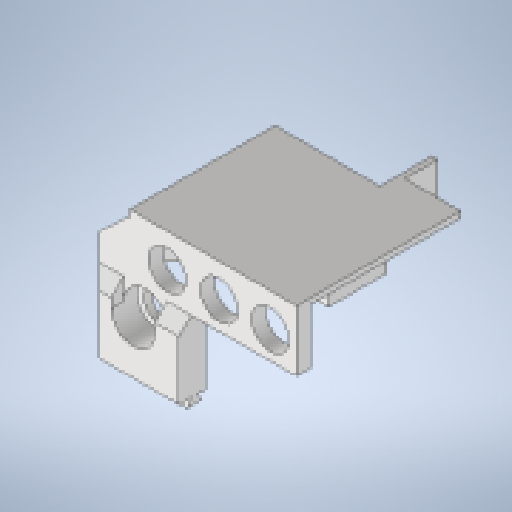
# Autodesk Inventor part: FrontLeftCover
Saved by Autodesk Inventor 2025.1 (Build 291241000, 241)
## iProperties
Created: 2026-04-16
Part Number: FrontLeftCover
Material: Generic
Document SubType Name: Modeling
Designer: User
Density: 1 g/cm^3
Appearance: Default
Author: User
## iProperties of the stored document FrontLeftCover_3DPrint.ipt
Created: 2026-04-17
Part Number: FrontLeftCover_3DPrint
Material: Generic
Document SubType Name: Modeling
Designer: User
Density: 1 g/cm^3
Appearance: Default
Author: User
Autodesk Inventor part; units mm, degrees
sketch "Sketch1" plane through (0, 0, 0) normal (0, 0, 1) x (1, 0, 0)
  line L0 (185.7556, 3.5) -> (29.0886, 3.5) projected
  line L1 (185.7556, 3.731) -> (29.0886, 3.731)
  line L2 (67.9918, 33.5) -> (67.9918, 28.504) projected
  line L3 (143.9918, 33.5) -> (67.9918, 33.5) projected
  line L4 (67.7918, 3.5) -> (67.7918, 33.7)
  line L5 (67.7918, 33.7) -> (143.9918, 33.7)
  line L6 (34.0886, 3.5) -> (34.0886, 0) projected
  line L7 (51.5977, 51.9) -> (63.6977, 51.9) projected
  line L8 (51.5977, 56.9) -> (63.6977, 56.9)
  line L9 (107.2766, 51.9) -> (107.2766, 38.5) projected
  line L10 (112.2766, 51.9) -> (112.2766, 38.5)
  line L11 (112.2766, 33.7) -> (112.2766, 56.9)
  line L12 (112.2766, 56.9) -> (34.0886, 56.9)
  line L13 (34.0886, 56.9) -> (34.0886, 3.731)
  line L14 (34.0886, 56.9) -> (29.0886, 56.9)
  line L15 (29.0886, 56.9) -> (29.0886, 3.731)
  circle A0 centre (57.6477, 45.2) radius 7.9 projected
  circle A1 centre (79.5677, 45.2) radius 7.9 projected
  circle A2 centre (101.2266, 45.2) radius 7.9 projected
  circle A3 centre (57.6477, 45.2) radius 8
  circle A4 centre (79.5677, 45.2) radius 8
  circle A5 centre (101.2266, 45.2) radius 8
  point P0 (0, 0)
  point P1 (29.0886, 3.5)
  point P2 (67.7918, 3.731)
  dimension "d0" = 0.231
  dimension "d1" = 0.2
  dimension "d2" = 5
  dimension "d3" = 5
  dimension "d4" = 0.1
  dimension "d5" = 0.1
  dimension "d6" = 0.1
  constraints: 20 end point, 5 point on line, 3 centre point, 2 parallel, 2 perpendicular, 1 horizontal, 2 other
  measures "d1" distance between parallel lines of L2 L4
  measures "d2" distance between parallel lines of L7 L8
  measures "d3" distance between parallel lines of L9 L10
  measures "d4" radial gap between concentric circles of A0 A3
  measures "d5" radial gap between concentric circles of A1 A4
  measures "d6" radial gap between concentric circles of A2 A5
ref_plane "Work Plane1" through (129.9918, 31.5, -11.1965) normal (0, 0, -1) x (0, 1, 0)
extrude "Extrusion1" add sketch "Sketch1" against normal up to surface (11.1965 mm away) contours L13 L12 L8 L11 L10 L5 L4 L1 | L1 L15 L14 L13
sketch "Sketch2" plane through (0, 0, 0) normal (0, 0, 1) x (1, 0, 0)
  circle A0 centre (57.6477, 45.2) radius 8 projected
  circle A1 centre (79.5677, 45.2) radius 8 projected
  circle A2 centre (101.2266, 45.2) radius 8 projected
  line L0 (112.2766, 56.9) -> (29.0886, 56.9) projected
  line L1 (112.2766, 33.7) -> (112.2766, 56.9) projected
  line L2 (67.7918, 33.7) -> (112.2766, 33.7) projected
  line L3 (29.0886, 56.9) -> (29.0886, 3.731) projected
  line L4 (67.7918, 3.731) -> (67.7918, 33.7) projected
  line L5 (112.2766, 56.9) -> (29.0886, 56.9)
  line L6 (29.0886, 56.9) -> (29.0886, 33.7)
  line L7 (29.0886, 33.7) -> (112.2766, 33.7)
  line L8 (112.2766, 33.7) -> (112.2766, 56.9)
  point P0 (0, 0)
  constraints: 8 end point, 2 parallel, 2 point on line, 1 horizontal, 1 perpendicular
ref_plane "Work Plane2" through (70.7677, 36.4, -5.1965) normal (0, 0, -1) x (0, 1, 0)
extrude "Extrusion2" cut sketch "Sketch2" against normal up to surface (5.1965 mm away)
sketch "Sketch3" plane through (0, 0, 0) normal (0, 0, 1) x (1, 0, 0)
  line L0 (67.7918, 33.7) -> (29.0886, 33.7) projected
  line L1 (29.0886, 33.7) -> (29.0886, 3.731) projected
  line L2 (29.0886, 3.731) -> (67.7918, 3.731) projected
  line L3 (67.7918, 3.731) -> (67.7918, 33.7) projected
  line L4 (34.0886, 28.7) -> (62.7918, 28.7)
  line L5 (62.7918, 28.7) -> (62.7918, 8.731)
  line L6 (62.7918, 8.731) -> (34.0886, 8.731)
  line L7 (34.0886, 8.731) -> (34.0886, 28.7)
  line L8 (48.4402, 24.5) -> (48.4402, 33.5)
  line L9 (29.0886, 33.7) -> (67.7918, 33.7) projected
  line L10 (29.0886, 33.7) -> (29.0886, 56.9) projected
  line L11 (48.4402, 33.7) -> (29.0886, 33.7)
  circle A0 centre (48.4402, 24.5) radius 9.2
  line L12 (48.4402, 33.5) -> (48.4402, 33.7)
  point P0 (0, 0)
  dimension "d11" = 5
  constraints: 14 end point, 2 vertical, 1 horizontal, 1 midpoint, 1 vertical alignment, 5 other
  measures "d11" distance between parallel lines of L0 L4
extrude "Extrusion3" cut sketch "Sketch3" against normal blind 11 contours A0 L4 L8 L12 | L12 L8 L4 A0 | A0 L4
sketch "Sketch4" plane through (112.2766, 56.9, -11.1965) normal (0, 0, -1) x (-1, 0, 0)
  circle A0 centre (63.8364, -32.4) radius 9.2 projected
  circle A1 centre (63.8364, -32.4) radius 6.5
  point P0 (112.2766, -56.9)
  dimension "d16" = 13
  constraints: 1 centre point, 1 coincident
  measures "d16" diameter of A1
extrude "Extrusion4" cut sketch "Sketch4" against normal blind 11 contours A1
sketch "Sketch5" plane through (112.2766, 56.9, -11.1965) normal (0, 0, -1) x (-1, 0, 0)
  circle A0 centre (63.8364, -32.4) radius 9.2 projected
  circle A1 centre (63.8364, -32.4) radius 6.5 projected
  point P0 (112.2766, -56.9)
  point P1 (63.8364, -23.2)
  constraints: 1 vertical alignment
extrude "Extrusion5" add sketch "Sketch5" along normal blind 3
sketch "Sketch6" plane through (0, 0, 0) normal (0, 0, 1) x (1, 0, 0)
  line L0 (48.4402, 33.7) -> (29.0886, 33.7) projected
  line L1 (67.7918, 33.7) -> (48.4402, 33.7) projected
  circle A0 centre (48.4402, 24.5) radius 9.2 projected
  line L2 (39.2402, 24.5) -> (39.2402, 33.7)
  line L3 (57.6402, 24.5) -> (57.6402, 33.7)
  point P0 (0, 0)
  constraints: 4 end point, 2 perpendicular, 2 point on circle, 2 point on line, 2 tangent
extrude "Extrusion6" cut sketch "Sketch6" against normal up to surface (5.1965 mm away) contours A0 L2 L0 | L1 L3 A0
chamfer "Chamfer2" distance 5.196 angle 45 2 edges at (34.1644, 33.7, 0) (62.716, 33.7, 0)
sketch "Sketch7" plane through (29.0886, 56.9, -11.1965) normal (0, 1, 0) x (1, 0, 0)
  line L0 (-29.0886, 22.8921) -> (-3, -3.1965) projected
  line L1 (0, -6.1965) -> (5, -11.1965) projected
  line L2 (2, -8.1965) -> (-5, -1.1965) projected
  line L3 (0, -11.1965) -> (10.1516, -11.1965) projected
  line L4 (0, -6.0005) -> (0, -11.1965) projected
  point P0 (-29.0886, -11.1965)
extrude "Extrusion7" cut sketch "Sketch7" against normal through all
sketch "Sketch8" plane through (29.0886, 3.731, -5) normal (-0.7071068, 0, 0.7071068) x (0.7071068, 0, 0.7071068)
  line L0 (7.0711, 24.773) -> (7.0711, 0) projected
  line L1 (7.0711, 0) -> (0, 0) projected
  line L2 (-41.1375, -3.731) -> (-41.1375, -0.231) projected
  line L3 (-52.5923, 2.269) -> (-42.7639, 2.269) projected
  line L4 (7.0711, 0) -> (30.9028, 0) projected
  line L5 (7.0711, 0) -> (-41.1375, 0)
  line L6 (-0.1389, 29.969) -> (-0.1389, 53.169) projected
  line L7 (-41.1375, 0) -> (-41.1375, 53.169)
  line L8 (-41.1375, 0) -> (12.0315, 0) construction
  line L9 (-41.1375, 53.169) -> (-0.1389, 53.169)
  line L10 (0, 29.773) -> (7.0711, 24.773) projected
  line L11 (-0.1386, 29.969) -> (0, 29.773) projected
  line L12 (-0.1386, 29.969) -> (-0.1389, 29.969) projected
  point P0 (-17.0332, -3.731)
  dimension "d31" = 90
  constraints: 8 end point, 2 horizontal, 2 perpendicular
  measures "d31" angle of L8 L7
extrude "Extrusion8" add sketch "Sketch8" against normal blind 5
sketch "Sketch9" plane through (0, 0, 0) normal (0, 0, 1) x (1, 0, 0)
  line L0 (28.9904, 56.9) -> (29.0886, 56.9) projected
  line L1 (28.9904, 56.9) -> (0, 56.9) projected
  line L2 (29.0886, 56.9) -> (112.2766, 56.9) projected
  circle A0 centre (57.6477, 45.2) radius 8.8 projected
  line L3 (0, 56.9) -> (0, 3.731) projected
  line L4 (0, 3.731) -> (34.0886, 3.731) projected
  line L5 (46.8477, 49.725) -> (46.8477, 40.675) projected
  line L6 (41.8477, 49.725) -> (41.8477, 40.675)
  line L7 (41.8477, 40.675) -> (41.8477, 56.9)
  line L8 (0, 3.731) -> (0, 6.731)
  line L9 (0, 6.731) -> (41.8477, 56.9)
  point P0 (0, 0)
  dimension "d34" = 5
  dimension "d35" = 3
  constraints: 8 end point, 2 point on line, 1 parallel, 1 vertical
  measures "d34" distance between parallel lines of L5 L6
  measures "d35" distance of L3.end L8.end
extrude "Extrusion9" cut sketch "Sketch9" against normal through all contours L0 L2 L9 L3 L1
sketch "Sketch12" plane through (67.7918, 3.731, -11.1965) normal (0, -1, 0) x (1, 0, 0)
  line L0 (-67.7918, -22.8921) -> (-64.2563, -26.4276) projected
  line L1 (-25.7956, -67.1884) -> (-67.7438, -25.2402) projected
  line L2 (-67.7438, -25.2402) -> (-63.0689, -25.2402)
  line L3 (-64.2563, -26.4276) -> (-37.8286, 0) projected
  line L4 (-67.7438, -25.2402) -> (-63.0689, -25.2402) construction
  line L5 (-68.1066, -24.2402) -> (-62.1095, -24.2402)
  line L6 (-62.5423, -24.2402) -> (-62.0689, -24.2402)
  point P0 (-67.7918, 11.1965)
  point P1 (-66.4437, -24.2402)
  dimension "d43" = 1
  constraints: 8 end point, 4 point on line, 2 horizontal, 1 collinear, 1 parallel
  measures "d43" distance between parallel lines of L5 L2
extrude "Extrusion10" cut sketch "Sketch12" against normal blind 10
sketch "Sketch13" plane through (0, 3.731, -34.0886) normal (-0.7071068, 0, -0.7071068) x (-0.7071068, 0, 0.7071068)
  line L0 (-1.9065, 4.6162) -> (-1.9065, 0) projected
  line L1 (0, 3) -> (0, 0) projected
  line L2 (0, 3) -> (-1.9065, 4.6162) projected
  line L3 (-11.5227, 2.269) -> (-1.6943, 2.269) projected
  line L4 (-14.3512, 2.269) -> (-11.5227, 2.269) projected
  line L5 (-14.3512, 2.269) -> (-57.8759, 2.269) projected
  line L6 (-57.8759, 3.269) -> (-14.3512, 3.269)
  line L7 (-14.3512, 3.269) -> (-11.5227, 3.269)
  line L8 (-11.5227, 3.269) -> (-1.6943, 3.269)
  line L9 (-57.8759, 5.769) -> (-14.3512, 5.769)
  line L10 (-14.3512, 5.769) -> (-11.5227, 5.769)
  line L11 (-11.5227, 5.769) -> (-1.6943, 5.769)
  line L12 (0, 37.755) -> (0, 3) projected
  line L13 (-1.6943, 5.769) -> (0, 5.769)
  line L14 (-1.6943, 3.269) -> (0, 3.269)
  line L15 (-46.8759, 2.269) -> (-46.8759, 6.269) projected
  line L16 (-45.8759, 2.269) -> (-45.8759, 6.269)
  point P0 (24.1043, -3.731)
  point P1 (-1.9065, 3.269)
  point P2 (-0.3173, 3.269)
  point P3 (-45.8759, 5.769)
  point P4 (-45.8759, 3.269)
  dimension "d46" = 1
  dimension "d47" = 2.5
  dimension "d48" = 1
  constraints: 18 end point, 2 perpendicular, 2 point on line, 1 parallel, 4 other
  measures "d46" distance between parallel lines of L5 L6
  measures "d47" distance between parallel lines of L6 L9
  measures "d48" distance between parallel lines of L15 L16
extrude "Extrusion11" add sketch "Sketch13" against normal blind 2.5 contours L0 L8 L7 L6 L16 L9 L10 L11 L13 L12 L14 L2
sketch "Sketch14" plane through (2.3097, 9.5, -35.4367) normal (0, 1, 0) x (1, 0, 0)
  line L0 (-2.3097, -1.3481) -> (30.1294, 31.091) projected
  line L1 (65.6821, 17.6568) -> (65.6821, 49.3641) projected
  line L2 (64.6821, 17.6568) -> (64.6821, 49.3641)
  line L3 (30.1294, 31.091) -> (64.6821, 31.091)
  line L4 (30.1294, 31.091) -> (64.6821, 31.091) construction
  line L5 (64.6821, 31.091) -> (64.6821, 28.591)
  line L6 (64.6821, 28.591) -> (27.6294, 28.591)
  point P0 (-2.3097, -35.4367)
  dimension "d51" = 1
  dimension "d52" = 0
  dimension "d53" = 2.5
  constraints: 10 end point, 3 point on line, 1 collinear, 1 horizontal, 1 parallel, 1 perpendicular
  measures "d51" distance between parallel lines of L1 L2
  measures "d52" distance between parallel lines of L3 L4
  measures "d53" distance of L4.end L5.end
extrude "Extrusion12" add sketch "Sketch14" against normal up to surface (2.5 mm away)
sketch "Sketch15" plane through (66.9918, 9.5, -66.5277) normal (0, 0, -1) x (-1, 0, 0)
  line L0 (0, 0) -> (0, -2.5) projected
  line L1 (-0.8, 24.2) -> (-45.2848, 24.2) projected
  line L2 (-0.8, 25.2) -> (-45.2848, 25.2)
  line L3 (0, -2.5) -> (0, 25.2)
  line L4 (0, 25.2) -> (-0.8, 25.2)
  line L5 (-23.6095, 43.606) -> (-23.6095, 36.106) projected
  line L6 (-21.6095, 43.606) -> (-21.6095, 36.106)
  line L7 (-26.6095, 55.106) -> (-23.6095, 55.106) projected
  line L8 (-26.6095, 57.106) -> (-23.6095, 57.106)
  line L9 (-21.6095, 25.2) -> (-21.6095, 57.106)
  line L10 (61.2689, -5.769) -> (61.2689, 4.092) projected
  line L11 (-21.6095, 57.106) -> (61.2689, 4.092)
  line L12 (34.5877, 0) -> (55.7465, 0) construction
  line L13 (0, 0) -> (34.5527, 0) projected
  line L14 (34.5527, 0) -> (34.5527, 21.1812)
  line L15 (34.5527, 0) -> (55.7339, 0) construction
  point P0 (66.9918, -9.5)
  point P1 (-21.6095, 43.606)
  point P2 (-21.6095, 36.106)
  dimension "d56" = 1
  dimension "d57" = 2
  dimension "d58" = 2
  dimension "d60" = 90
  constraints: 20 end point, 3 parallel, 2 horizontal, 2 perpendicular, 2 point on line, 2 vertical
  measures "d56" distance between parallel lines of L1 L2
  measures "d57" distance between parallel lines of L5 L6
  measures "d58" distance between parallel lines of L7 L8
  measures "d60" angle of L15 L14
extrude "Extrusion13" add sketch "Sketch15" against normal blind 2.5
sketch "Sketch16" plane through (0, 3.731, -34.0886) normal (-0.7071068, 0, -0.7071068) x (-0.7071068, 0, 0.7071068)
  line L0 (-45.8759, 5.769) -> (-45.8759, 26.9502) projected
  line L1 (-5, 9.861) -> (-2.5865, 5.769) projected
  line L2 (0, 5.769) -> (-45.8759, 5.769) projected
  line L3 (-45.8759, 26.9502) -> (-5, 9.861)
  point P0 (24.1043, -3.731)
  constraints: 2 end point
extrude "Extrusion14" add sketch "Sketch16" against normal blind 2.5
ref_plane "Work Plane3" through (41.8477, 56.9, -5.1965) normal (0.6694405, -0.7146449, 0.2028105) x (-0.6019698, -0.6818384, -0.4156065)
sketch "Sketch18" plane through (41.8477, 56.9, -5.1965) normal (0.6694405, -0.7146449, 0.2028105) x (-0.6019698, -0.6818384, -0.4156065)
  line L0 (71.2225, -0.3903) -> (69.5179, 0) projected
  line L1 (49.0303, 46.1898) -> (69.5179, 0)
  line L2 (69.5179, 0) -> (0, 0)
  line L3 (49.0303, 46.1898) -> (-9.2725, 76.2461) projected
  line L4 (0, 0) -> (49.0303, 46.1898)
  point P0 (61.828, -31.7078)
  constraints: 6 end point, 1 horizontal
extrude "Extrusion15" add sketch "Sketch18" along normal blind 2.5
sketch "Sketch19" plane through (0, 9.5, -34.0886) normal (-0.4352951, -0.156138, 0.8866449) x (0.6019698, 0.6818384, 0.4156065)
  line L0 (1.5874, 0) -> (3.449, 1.2745) projected
  line L1 (3.449, 1.2745) -> (4.9358, 0) projected
  line L2 (3.449, 1.2745) -> (20.4876, 0) projected
  line L3 (69.5179, 0) -> (0, 0) projected
  line L4 (57.8032, 0) -> (67.0243, 1.2169) projected
  line L5 (67.0243, 1.2169) -> (69.5179, 0) projected
  point P0 (7.69, -13.7027)
extrude "Extrusion16" cut sketch "Sketch19" against normal through all
sketch "Sketch20" plane through (0, 9.5, -34.0886) normal (-0.4352951, -0.156138, 0.8866449) x (0.6019698, 0.6818384, 0.4156065)
  line L0 (31.6827, -2.5) -> (35.7207, -0.8873) projected
  line L1 (53.8612, -2.5) -> (31.6827, -2.5) projected
  line L2 (54.8939, -0.3839) -> (53.8612, -2.5) projected
  line L3 (69.5179, 0) -> (54.8939, -0.3839) projected
  line L4 (69.5179, 0) -> (0, 0) projected
  line L5 (1.8617, -1.7762) -> (0, 0) projected
  line L6 (35.7207, -0.8873) -> (1.8617, -1.7762) projected
  line L7 (51.3092, -2.4282) -> (1.3558, -2.0063) projected
  line L8 (1.7988, -1.5419) -> (1.3558, -2.0063) projected
  point P0 (7.69, -13.7027)
  point P1 (1.7118, -1.6332)
  point P2 (32.2652, -2.2674)
extrude "Extrusion17" add sketch "Sketch20" along normal up to surface surface through (29.0886, 56.9, -5) normal (0.7071068, 0, -0.7071068)
sketch "Sketch21" plane through (112.2766, 56.9, -5.1965) normal (0, 1, 0) x (1, 0, 0)
  line L0 (-70.4289, 0) -> (0, 0) projected
  line L1 (-70.4289, 0) -> (-74.695, -8.6895) projected
  line L2 (-74.695, -8.6895) -> (-112.2766, 28.8921) projected
  line L3 (-62.6289, 0) -> (-46.6289, 0) projected
  line L4 (-83.188, 0) -> (-73.0364, 0) projected
  line L5 (-60.1795, 0) -> (-83.188, 0)
  line L6 (-68.6111, 6) -> (-70.4289, 0) projected
  line L7 (-70.4289, 0) -> (-83.3845, 0)
  point P0 (-112.2766, -5.1965)
  constraints: 4 end point, 3 point on line, 1 horizontal
extrude "Extrusion18" cut sketch "Sketch21" against normal up to surface surface through (91.4796, 31.102, -2.598) normal (0, 0.7071068, 0.7071068)
sketch "Sketch22" plane through (67.7918, 33.7, -5.1965) normal (0, 0, 1) x (1, 0, 0)
  line L0 (-37.436, 11.8978) -> (-36.8153, 10.1671) projected
  line L1 (-25.9441, 23.2) -> (-37.436, 11.8978) projected
  line L2 (-25.9441, 23.2) -> (-36.8153, 10.1671) projected
  point P0 (-67.7918, -33.7)
extrude "Extrusion19" add sketch "Sketch22" against normal up to surface surface through (33.3015, 46.6544, -11.1965) normal (0.6850081, -0.6965045, 0.2136479)
sketch "Sketch23" plane through (112.2766, 56.9, -5.1965) normal (0, 1, 0) x (1, 0, 0)
  line L0 (-70.4289, 0) -> (-68.7553, -0.507) projected
  line L1 (-68.8331, 0) -> (-68.7553, -0.507) projected
  line L2 (-70.4289, 0) -> (0, 0) projected
  point P0 (-112.2766, -5.1965)
extrude "Extrusion20" cut sketch "Sketch23" against normal blind 10
sketch "Sketch24" plane through (112.2766, 56.9, -5.1965) normal (0, 1, 0) x (1, 0, 0)
  line L0 (0, 0) -> (0, 6) projected
  line L1 (-70.4289, 0) -> (0, 0) projected
  line L2 (-38.7589, 41.9) -> (-26.6589, 41.9) projected
  line L3 (-38.7589, 56.9) -> (-26.6589, 56.9)
  line L4 (0, 0) -> (-70.4289, 0)
  line L5 (-79.8375, 61.3312) -> (-23.6753, 61.3312) projected
  line L6 (-70.4289, 0) -> (0, 0)
  line L7 (0, 0) -> (0, 61.3312)
  line L8 (0, 61.3312) -> (-70.4289, 61.3312)
  line L9 (-70.4289, 61.3312) -> (-70.4289, 0)
  point P0 (-112.2766, -5.1965)
  point P1 (-70.4289, 61.3312)
  point P2 (-23.6753, 61.3312)
  dimension "d33" = 0
  dimension "d77" = 15
  constraints: 12 end point, 3 parallel, 2 horizontal, 1 perpendicular
  measures "d77" distance between parallel lines of L2 L3
extrude "Extrusion21" add sketch "Sketch24" along normal blind 2.5
sketch "Sketch25" plane through (66.9918, 7, -66.5277) normal (0, 0, -1) x (-1, 0, 0)
  line L0 (-6.4358, 49.9) -> (25.1441, 49.9) projected
  line L1 (34.5527, 23.6812) -> (-6.4358, 49.9) projected
  line L2 (38.0997, 37.7639) -> (25.1441, 49.9) projected
  line L3 (25.1441, 49.9) -> (22.6441, 49.9)
  line L4 (22.6441, 49.9) -> (22.6441, 31.2987)
  point P0 (66.9918, -7)
  dimension "d80" = 2.5
  constraints: 4 end point, 2 point on line, 1 perpendicular
  measures "d80" distance of L0.end L3.end
extrude "Extrusion22" add sketch "Sketch25" against normal blind 2.5
sketch "Sketch26" plane through (66.9918, 7, -66.5277) normal (0, 0, -1) x (-1, 0, 0)
  line L0 (22.6441, 49.9) -> (25.1441, 49.9) projected
  line L1 (22.6441, 31.2987) -> (22.6441, 49.9) projected
  line L2 (34.5527, 23.6812) -> (22.6441, 31.2987) projected
  line L3 (25.1441, 49.9) -> (25.1441, 52.4) projected
  line L4 (25.1441, 49.9) -> (25.1441, 29.6995)
  point P0 (66.9918, -7)
  constraints: 2 end point, 1 collinear, 1 point on line
extrude "Extrusion23" add sketch "Sketch26" against normal up to surface surface through (32.4391, 30.6812, -66.5277) normal (0.7296167, 0.5811913, -0.3603834)
sketch "Sketch27" plane through (40.9273, 54.335, -11.1965) normal (0.7296167, 0.5811913, -0.3603834) x (-0.1396745, -0.3892292, -0.9104898)
  line L0 (-6.5899, 0) -> (-0.4642, 0) projected
  line L1 (0, 0) -> (-0.4642, 0) projected
  line L2 (60.7709, 0) -> (0, 0) projected
  line L3 (45.3092, 0) -> (60.7709, 0) projected
  line L4 (44.0106, 0) -> (45.3092, 0) projected
  line L5 (-0.0566, 0) -> (44.0106, 0) projected
  line L6 (-0.0566, 0) -> (-6.5899, 0) projected
  line L7 (0.3212, -1.4419) -> (5.3923, -2.5) projected
  line L8 (58.5819, -2.5) -> (5.3923, -2.5) projected
  line L9 (58.1767, -0.6807) -> (58.5819, -2.5) projected
  line L10 (60.7709, 0) -> (58.1767, -0.6807) projected
  line L11 (60.7709, 0) -> (0, 0) projected
  line L12 (0.3212, -1.4419) -> (0, 0) projected
  line L13 (-6.5899, 0) -> (-0.4642, 0) projected
  line L14 (-0.4642, 0) -> (0.3212, -1.4419) projected
  point P0 (16.671, -13.7027)
  point P1 (60.7709, 0)
extrude "Extrusion24" add sketch "Sketch27" along normal blind 14.5
sketch "Sketch28" plane through (43.5213, 55.1134, -4.6895) normal (0.6694405, -0.7146449, 0.2028105) x (0.6019698, 0.6818384, 0.4156065)
  line L0 (-38.2241, -49.0084) -> (-27.3128, -25.7305) projected
  line L1 (-27.3128, -25.7305) -> (-21.5421, -20.2941) projected
  line L2 (-21.5421, -20.2941) -> (-5.6654, -5.3372) projected
  line L3 (-35.118, -50.4632) -> (-6.372, -10.7103) projected
  line L4 (-35.6288, -50.3463) -> (-38.2241, -49.0084) projected
  line L5 (-23.1287, -8.3115) -> (-2.6947, -12.9908) projected
  line L6 (-35.118, -50.4632) -> (-35.6288, -50.3463) projected
  line L7 (-33.3168, -51.3076) -> (-35.118, -50.4632) projected
  line L8 (-38.2464, -48.9969) -> (-48.608, -44.14) projected
  line L9 (-38.2241, -49.0084) -> (-38.2464, -48.9969) projected
  point P0 (-61.828, 31.7078)
  point P1 (-7.2644, -11.9444)
  point P2 (-11.6201, -10.9469)
extrude "Extrusion25" cut sketch "Sketch28" along normal blind 14.5
sketch "Sketch29" plane through (44.3477, 42.2304, -64.0277) normal (1, 0, 0) x (0, 0, -1)
  line L0 (-52.8312, 14.6696) -> (2.5, 14.6696) projected
  line L1 (0, -7.5304) -> (0, 14.6696) projected
  line L2 (-52.8312, -8.5304) -> (-52.8312, 14.6696) projected
  line L3 (-52.8312, 14.6696) -> (0, 14.6696)
  line L4 (0, 14.6696) -> (0, -7.5304)
  line L5 (0, -7.5304) -> (-52.8312, -7.5304)
  line L6 (-52.8312, -7.5304) -> (-52.8312, 14.6696)
  point P0 (-64.0277, -42.2304)
  constraints: 8 end point, 2 parallel, 1 horizontal, 1 perpendicular
extrude "Extrusion26" cut sketch "Sketch29" along normal blind 14.5
sketch "Sketch31" plane through (43.5213, 55.1134, -4.6895) normal (0.6694405, -0.7146449, 0.2028105) x (0.6019698, 0.6818384, 0.4156065)
  line L0 (-7.2644, -11.9444) -> (-10.8274, -11.1285) projected
  line L1 (-10.8274, -11.1285) -> (-11.6201, -10.9469) projected
  line L2 (-8.7215, -8.2163) -> (-11.6201, -10.9469) projected
  line L3 (-8.7215, -8.2163) -> (-5.2019, -4.9006) projected
  line L4 (-0.9887, -6.4081) -> (-22.9457, -53.2507) projected
  line L5 (39.9024, -35.9772) -> (-0.9887, -6.4081) projected
  line L6 (-5.2019, -4.9006) -> (-5.6654, -5.3372) projected
  line L7 (-5.6654, -5.3372) -> (-0.9887, -6.4081) projected
  line L8 (-20.7848, 2.4037) -> (-5.2019, -4.9006) projected
  line L9 (-11.6201, -10.9469) -> (-3.9406, -12.7055)
  line L10 (-3.9406, -12.7055) -> (-0.9887, -6.4081)
  line L11 (-5.2019, -4.9006) -> (-11.6201, -10.9469)
  line L12 (-11.0625, -2.1535) -> (-1.1683, -6.7913)
  point P0 (-61.828, 31.7078)
  point P1 (-1.1683, -6.7913)
  point P2 (-5.2019, -4.9006)
  point P3 (-7.2644, -11.9444)
  point P4 (-3.9406, -12.7055)
  constraints: 8 end point, 3 point on line, 2 collinear
extrude "Extrusion27" cut sketch "Sketch31" against normal up to surface contours L0 L1 L2 L3 L7 L12 L4 L9 | L7 L3 L12 surface through (70.6826, 30.3155, -11.1965) normal (0, 0, -1)
sketch "Sketch32" plane through (112.2766, 59.4, -5.1965) normal (0, 1, 0) x (1, 0, 0)
  line L0 (-34.9406, 61.3312) -> (-70.4289, 61.3312) projected
  line L1 (-59.6181, 61.3312) -> (-88.0349, 61.3312)
  line L2 (-88.0349, 61.3312) -> (-88.0349, 76.9498)
  line L3 (-88.0349, 76.9498) -> (-59.6181, 76.9498)
  line L4 (-59.6181, 76.9498) -> (-59.6181, 61.3312)
  point P0 (-112.2766, -5.1965)
  point P1 (-70.4289, 61.3312)
  constraints: 8 end point, 2 parallel, 1 horizontal, 1 perpendicular, 1 point on line
extrude "Extrusion28" cut sketch "Sketch32" against normal through all
sketch "Sketch33" plane through (66.9918, 7, -66.5277) normal (0, 0, -1) x (-1, 0, 0)
  line L0 (34.5527, 23.6812) -> (28.6733, 28.2363) projected
  line L1 (34.5527, 23.6812) -> (28.2542, 27.7102) projected
  line L2 (28.6733, 28.2363) -> (28.2542, 27.7102) projected
  point P0 (66.9918, -7)
extrude "Extrusion29" add sketch "Sketch33" along normal up to surface surface through (34.4185, 29.7466, -64.0277) normal (-0.2818831, -0.2245398, -0.9328043)
sketch "Sketch34" plane through (112.2766, 59.4, -5.1965) normal (0, 1, 0) x (1, 0, 0)
  line L0 (-70.4289, 0) -> (0, 0) projected
  line L1 (-63.8114, 0) -> (-74.8638, 0)
  line L2 (-74.8638, 0) -> (-74.8638, -8.063)
  line L3 (-74.8638, -8.063) -> (-63.8114, -8.063)
  line L4 (-63.8114, -8.063) -> (-63.8114, 0)
  point P0 (-112.2766, -5.1965)
  point P1 (-70.4289, 0)
  constraints: 8 end point, 2 parallel, 1 horizontal, 1 perpendicular, 1 point on line
extrude "Extrusion30" cut sketch "Sketch34" against normal blind 10
sketch "Sketch35" plane through (41.8477, 39.4947, -66.5277) normal (-1, 0, 0) x (0, 0, 1)
  line L0 (0, 19.9053) -> (61.3312, 19.9053) projected
  line L1 (-10.2184, 45.465) -> (63.5572, 45.465)
  line L2 (63.5572, 45.465) -> (63.5572, 19.9053)
  line L3 (63.5572, 19.9053) -> (-10.2184, 19.9053)
  line L4 (-10.2184, 19.9053) -> (-10.2184, 45.465)
  point P0 (66.5277, -39.4947)
  point P1 (0, 19.9053)
  point P2 (61.3312, 19.9053)
  constraints: 8 end point, 2 parallel, 1 horizontal, 1 perpendicular
extrude "Extrusion31" cut sketch "Sketch35" against normal through all
sketch "Sketch36" plane through (0, 3.731, -34.0886) normal (-0.7071068, 0, -0.7071068) x (-0.7071068, 0, 0.7071068)
  line L0 (-2.5865, 5.769) -> (-3.5544, 7.4101) projected
  line L1 (0, 5.769) -> (-2.5865, 5.769) projected
  line L2 (0, 5.769) -> (-3.5544, 7.4101) projected
  point P0 (24.1043, -3.731)
extrude "Extrusion32" add sketch "Sketch36" against normal up to surface surface through (0, 9.5, -34.0886) normal (-0.3737746, -0.5599702, -0.7394092)
sketch "Sketch37" plane through (0, 3.731, -34.0886) normal (-0.7071068, 0, -0.7071068) x (-0.7071068, 0, 0.7071068)
  line L0 (0, 5.769) -> (-45.8759, 26.9502) projected
  line L1 (-45.8759, 26.9502) -> (-45.8759, 3.269) projected
  line L2 (-45.8759, 3.269) -> (-1.9065, 3.269) projected
  line L3 (-1.9065, 3.269) -> (-1.9065, 0) projected
  line L4 (0, 0) -> (-1.9065, 0) projected
  line L5 (0, 3) -> (0, 0) projected
  line L6 (0, 3) -> (-0.3173, 3.269) projected
  line L7 (-0.3173, 3.269) -> (0, 3.269) projected
  line L8 (0, 3.269) -> (0, 5.769) projected
  line L9 (-0.3173, 3.269) -> (0, 3.269) projected
  line L10 (0, 3.269) -> (0, 3) projected
  point P0 (24.1043, -3.731)
extrude "Extrusion33" add sketch "Sketch37" along normal up to surface contours L10 L6 L7 surface through (41.8477, 56.9, 0) normal (0.7679186, -0.6405475, 0)
chamfer "Chamfer3" distance 3 angle 45 1 edges at (57.6402, 24.5, -11.1965)
sketch "Sketch38" plane through (5.723, 3.731, -35.4367) normal (0, 0, -1) x (-1, 0, 0)
  line L0 (0.8393, 6.4629) -> (0, 7.2491) projected
  line L1 (0, 0) -> (0, 7.2491) projected
  line L2 (0.8393, 3.269) -> (0.8393, 6.4629) projected
  line L3 (4.3749, 3.269) -> (0.8393, 3.269) projected
  line L4 (4.3749, 3.269) -> (0, 3.269)
  line L5 (-26.7162, 3.269) -> (4.3749, 3.269) projected
  point P0 (5.723, -3.731)
  constraints: 2 end point, 2 point on line
extrude "Extrusion34" add sketch "Sketch38" along normal up to surface surface through (17.9873, 8.25, -48.5404) normal (0.7071068, 0, 0.7071068)
sketch "Sketch39" plane through (67.7918, 3.731, -11.1965) normal (1, 0, 0) x (0, 0, -1)
  line L0 (-8.1965, -3.231) -> (-6.1965, -0.231) projected
  line L1 (-1.1965, -3.231) -> (-8.1965, -3.231) projected
  line L2 (-3.1965, -0.231) -> (-1.1965, -3.231) projected
  line L3 (-6.0193, -0.3492) -> (-7.7985, -3.018)
  line L4 (-7.7985, -3.018) -> (-1.5945, -3.018)
  line L5 (-1.5945, -3.018) -> (-3.3737, -0.3492)
  line L6 (-11.1965, 0) -> (0, 0) projected
  line L7 (-7.7985, -3.018) -> (-5.7865, 0)
  line L8 (-1.5945, -3.018) -> (-3.6065, 0)
  point P0 (-11.1965, -3.731)
  point P1 (-3.3737, -0.3492)
  point P2 (-6.0193, -0.3492)
  dimension "d110" = 0.213
  constraints: 10 end point, 4 point on line, 2 other
  measures "d110" distance between parallel lines of L0 L3
extrude "Extrusion35" add sketch "Sketch39" against normal up to surface surface through (29.0886, 56.9, -5) normal (0.7071068, 0, -0.7071068)
sketch "Sketch40" plane through (66.9918, 7, -66.5277) normal (0, 0, -1) x (-1, 0, 0)
  line L0 (-21.6095, 49.9) -> (-21.6095, 27.7) projected
  line L1 (-21.6095, 27.7) -> (0, 27.7) projected
  line L2 (-45.2848, 52.4) -> (25.1441, 52.4) projected
  line L3 (-21.6095, 27.7) -> (-19.1095, 27.7)
  line L4 (-19.1095, 27.7) -> (-19.1095, 52.4)
  line L5 (-19.1095, 52.4) -> (-21.6095, 52.4)
  line L6 (-21.6095, 52.4) -> (-21.6095, 27.7)
  point P0 (66.9918, -7)
  point P1 (-21.6095, 52.4)
  dimension "d113" = 2.5
  constraints: 8 end point, 2 parallel, 1 horizontal, 1 perpendicular, 1 point on line
  measures "d113" distance of L5.end L4.end
ref_plane "Work Plane4" through (94.3013, 43.856, -88.3598) normal (0, 0, -1) x (0, 1, 0)
extrude "Extrusion36" add sketch "Sketch40" along normal up to surface (21.832 mm away)
sketch "Sketch41" plane through (112.2766, 59.4, -5.1965) normal (0, 1, 0) x (1, 0, 0)
  line L0 (-23.6753, 61.3312) -> (-23.6753, 83.1633) projected
  line L1 (0, 61.3312) -> (-23.6753, 61.3312) projected
  line L2 (0, 0) -> (0, 61.3312) projected
  line L3 (-18.5753, 69.2633) -> (66.4247, 69.2633) projected
  line L4 (-23.6753, 61.3312) -> (0, 61.3312)
  line L5 (0, 61.3312) -> (0, 69.2633)
  line L6 (0, 69.2633) -> (-23.6753, 69.2633)
  line L7 (-23.6753, 69.2633) -> (-23.6753, 61.3312)
  point P0 (-112.2766, -5.1965)
  constraints: 8 end point, 2 parallel, 1 horizontal, 1 perpendicular, 1 point on line
extrude "Extrusion37" add sketch "Sketch41" against normal up to surface (2.5 mm away)
sketch "Sketch42" plane through (86.1013, 34.7, -66.5277) normal (-1, 0, 0) x (0, 0, 1)
  line L0 (0, 24.7) -> (0, 0) projected
  line L1 (0, 0) -> (-21.832, 0) projected
  line L2 (-21.832, 24.7) -> (-21.832, 0) projected
  line L3 (2.5, 0) -> (-21.832, 0) projected
  line L4 (-21.832, 0) -> (-21.832, 2.5)
  line L5 (-21.832, 2.5) -> (0, 2.5)
  point P0 (66.5277, -34.7)
  dimension "d118" = 2.5
  constraints: 4 end point, 2 point on line, 1 perpendicular
  measures "d118" distance of L1.end L4.end
extrude "Extrusion38" add sketch "Sketch42" along normal up to surface (19.1095 mm away)
sketch "Sketch43" plane through (66.9918, 34.7, -88.3598) normal (-1, 0, 0) x (0, 0, 1)
  line L0 (21.832, 2.5) -> (0, 2.5) projected
  line L1 (21.832, 0) -> (21.832, -27.7) projected
  line L2 (21.832, 2.5) -> (21.832, 0) projected
  line L3 (21.832, 2.5) -> (0, 2.5)
  line L4 (0, 2.5) -> (0, -27.7)
  line L5 (0, -27.7) -> (21.832, -27.7)
  line L6 (21.832, -27.7) -> (21.832, 2.5)
  point P0 (88.3598, -34.7)
  point P1 (21.832, -27.7)
  constraints: 8 end point, 2 parallel, 1 horizontal, 1 perpendicular
extrude "Extrusion39" add sketch "Sketch43" along normal blind 2.5
sketch "Sketch44" plane through (67.7918, 3.731, -11.1965) normal (1, 0, 0) x (0, 0, -1)
  line L0 (-11.1965, 0) -> (-11.1965, 24.773) projected
  line L1 (-11.1965, -0.231) -> (-6.1965, -0.231) projected
  line L2 (0, 0) -> (0, 29.969) projected
  line L3 (-8.6965, 0) -> (-8.6965, 24.773)
  line L4 (-2.5, 0) -> (-2.5, 29.969)
  line L5 (-8.6965, 24.773) -> (-2.5, 24.773)
  line L6 (-8.6965, 0) -> (-8.6965, 2.5)
  line L7 (-8.6965, 2.5) -> (-2.5, 2.5)
  point P0 (-11.1965, -3.731)
  dimension "d123" = 2.5
  dimension "d124" = 2.5
  dimension "d125" = 2.5
  constraints: 10 end point, 3 point on line, 2 parallel, 2 perpendicular
  measures "d123" distance between parallel lines of L0 L3
  measures "d124" distance between parallel lines of L2 L4
  measures "d125" distance of L3.start L6.end
extrude "Extrusion40" cut sketch "Sketch44" against normal blind 7
sketch "Sketch45" plane through (64.4918, 34.7, -88.3598) normal (-1, 0, 0) x (0, 0, 1)
  line L0 (-5.5815, -24.7) -> (4.4185, -24.7) projected
  line L1 (4.4185, -24.7) -> (19.9749, -24.7) projected
  line L2 (19.9749, -28.7) -> (19.9749, -24.7) projected
  line L3 (21.4749, -28.7) -> (21.4749, -23.2)
  line L4 (21.4749, -23.2) -> (4.4185, -23.2)
  line L5 (4.4185, -23.2) -> (-5.5815, -23.2)
  line L6 (0, 2.5) -> (0, -27.7) projected
  line L7 (0, -27.7) -> (21.832, -27.7) projected
  line L8 (0, -23.2) -> (21.832, -23.2)
  line L9 (21.832, -23.2) -> (21.832, -27.7)
  line L10 (21.832, -27.7) -> (0, -27.7)
  line L11 (0, -27.7) -> (0, -23.2)
  point P0 (88.3598, -34.7)
  dimension "d128" = 1.5
  constraints: 14 end point, 2 parallel, 2 point on line, 1 horizontal, 1 perpendicular, 2 other
  measures "d128" distance between parallel lines of L1 L4
extrude "Extrusion41" cut sketch "Sketch45" against normal blind 7
sketch "Sketch46" plane through (86.1013, 37.2, -66.5277) normal (0, 1, 0) x (1, 0, 0)
  line L0 (0, 0) -> (0, 21.832) projected
  line L1 (0, 0) -> (-44.2536, 0) projected
  line L2 (0, 0) -> (-5, 0)
  line L3 (-5, 0) -> (-5, 5)
  line L4 (-5, 5) -> (0, 5)
  line L5 (0, 5) -> (0, 0)
  circle A0 centre (-5, 5) radius 1.5
  point P0 (-86.1013, -66.5277)
  dimension "d131" = 5
  dimension "d132" = 5
  dimension "d133" = 3
  constraints: 8 end point, 2 parallel, 1 centre point, 1 coincident, 1 horizontal, 1 perpendicular
  measures "d131" distance of L3.end L4.end
  measures "d132" distance of L2.end L3.end
  measures "d133" diameter of A0
extrude "Extrusion42" cut sketch "Sketch46" against normal blind 7 contours A0 L3 L4 | L4 L3 A0
sketch "Sketch47" plane through (112.2766, 33.7, -5.1965) normal (1, 0, 0) x (0, 0, -1)
  line L0 (0, 25.7) -> (69.2633, 25.7) projected
  line L1 (0, 25.7) -> (0, 0) projected
  line L2 (0, 0) -> (6, 0) projected
  line L3 (69.2633, 25.7) -> (69.2633, 23.2) projected
  line L4 (6, 0) -> (6, 23.2) projected
  line L5 (69.2633, 23.2) -> (58.8312, 23.2) projected
  line L6 (6, 0) -> (69.2633, 23.2)
  point P0 (-5.1965, -33.7)
  constraints: 2 end point
extrude "Extrusion43" add sketch "Sketch47" along normal blind 2.5
body "Solid1"
